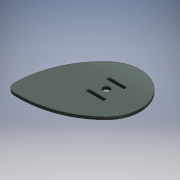
# Autodesk Inventor part: leva00
Saved by Autodesk Inventor 2016 (Build 200138000, 138)
## iProperties
Created: 2016-09-20
Part Number: leva00
Material: Madera (abedul)
Document SubType Name: Modeling
Designer: i95sa
Density: 0.55 g/cm^3
Appearance: Gris plomo - Pulido
Author: i95sa
Autodesk Inventor part; units mm, degrees
ref_plane "YZ Plane" through (0, 0, 0) normal (1, 0, 0) x (0, 1, 0)
ref_plane "XZ Plane" through (0, 0, 0) normal (0, 1, 0) x (-1, 0, 0)
ref_plane "XY Plane" through (0, 0, 0) normal (0, 0, 1) x (1, 0, 0)
sketch "Boceto1" plane through (0, 0, 0) normal (0, 0, 1) x (1, 0, 0)
  arc A0 (35.4425, 33.2827) -> (-35.4425, -33.2827) centre (0, 0) ccw
  arc A1 (-54.5431, -51.2194) -> (-70.9012, -66.5807) centre (-62.7222, -58.9) ccw
  line L0 (-73.2692, -68.8044) -> (-80.9499, -60.6254)
  line L1 (-32.8605, 35.8342) -> (-45.6615, 49.4659)
  line L2 (-45.6615, 49.4659) -> (-80.9499, -60.6254)
  line L3 (-80.9499, -60.6254) -> (-67.2507, -17.8872)
  arc A2 (-32.8605, 35.8342) -> (-67.2507, -17.8872) centre (51.2282, -55.8641) ccw
  arc A3 (-67.2507, -17.8872) -> (-73.941, -58.7376) centre (66.5387, -60.7717) ccw
  line L4 (2.7263, 2.5602) -> (35.4425, 33.2827)
  line L5 (-2.7263, -2.5602) -> (-73.2692, -68.8044)
  arc A4 (-35.4425, -33.2827) -> (35.4425, 33.2827) centre (0, 0) ccw
  arc A5 (-70.9012, -66.5807) -> (-54.5431, -51.2194) centre (-62.7222, -58.9) ccw
  line L6 (-73.2692, -68.8044) -> (-65.5886, -76.9834)
  line L7 (33.7002, -35.0457) -> (46.5012, -48.6774)
  line L8 (46.5012, -48.6774) -> (-65.5886, -76.9834)
  line L9 (-65.5886, -76.9834) -> (-22.0747, -65.9949)
  arc A6 (-22.0747, -65.9949) -> (33.7002, -35.0457) centre (-52.5372, 54.6348) ccw
  arc A7 (-63.2645, -70.1069) -> (-22.0747, -65.9949) centre (-56.4738, 70.2233) ccw
  dimension "d0" = 97.24
  dimension "d6" = 22.44
  dimension "d7" = 11.22
  dimension "d8" = 18.7
  dimension "d9" = 44.88
  constraints: 20 end point, 20 point on circle, 8 centre point, 6 symmetric about line, 5 point on line, 4 tangent, 1 collinear, 4 other
  measures "d0" diameter of A0
  measures "d6" diameter of A1
  measures "d7" distance of L0.start L0.end
  measures "d8" distance of L1.start L1.end
  measures "d9" distance of L0.end L3.end
extrude "Extrusión2" add sketch "Boceto1" along normal blind 4 contours A4 A0 | A0 L5 A1 A3 A2 | A6 A7 A5 L5 A4 | L5 A1 | A5 L5
sketch "Boceto2" plane through (0, 0, 4) normal (0, 0, 1) x (1, 0, 0)
  line L0 (0, 0) -> (0, 12.5)
  line L1 (0, 12.5) -> (-12.5, 12.5)
  line L2 (-12.5, 12.5) -> (-12.5, 16.7)
  line L3 (-12.5, 16.7) -> (12.5, 16.7)
  line L4 (12.5, 16.7) -> (12.5, 12.5)
  line L5 (12.5, 12.5) -> (0, 12.5)
  line L6 (0, 0) -> (12.5, 0)
  line L7 (0, 0) -> (0, -12.5)
  line L8 (0, -12.5) -> (-12.5, -12.5)
  line L9 (-12.5, -12.5) -> (-12.5, -16.7)
  line L10 (-12.5, -16.7) -> (12.5, -16.7)
  line L11 (12.5, -16.7) -> (12.5, -12.5)
  line L12 (12.5, -12.5) -> (0, -12.5)
  circle A0 centre (0, 0) radius 5
  dimension "d24" = 12.5
  dimension "d25" = 12.5
  dimension "d26" = 4.2
  dimension "d27" = 25
  dimension "d28" = 10
  constraints: 26 end point, 5 perpendicular, 5 symmetric about line, 3 point on line, 1 centre point, 1 coincident, 1 parallel, 1 vertical
  measures "d24" distance of L0.start L0.end
  measures "d25" distance of L0.end L1.end
  measures "d26" distance of L1.end L2.end
  measures "d27" distance of L2.end L3.end
  measures "d28" diameter of A0
extrude "Extrusión3" cut sketch "Boceto2" against normal blind 4
